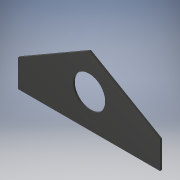
# Autodesk Inventor part: CA01
Saved by Autodesk Inventor 2017 (Build 210142000, 142)
## iProperties
Created: 2019-03-26
Part Number: CA01
Material: ABS Plastic
Document SubType Name: Modeling
Designer: Dell
Density: 1.06 g/cm^3
Appearance: Smooth - Black
Author: Dell
Autodesk Inventor part; units mm, degrees
ref_plane "YZ Plane" through (0, 0, 0) normal (1, 0, 0) x (0, 1, 0)
ref_plane "XZ Plane" through (0, 0, 0) normal (0, 1, 0) x (-1, 0, 0)
ref_plane "XY Plane" through (0, 0, 0) normal (0, 0, 1) x (1, 0, 0)
sketch "Sketch1" plane through (0, 0, 0) normal (0, 0, 1) x (1, 0, 0)
  line L0 (0, 0) -> (525.78, 0)
  line L1 (0, 0) -> (0, 101.6)
  line L2 (0, 101.6) -> (262.89, 253.3796)
  line L3 (262.89, 253.3796) -> (525.78, 101.6)
  line L4 (525.78, 101.6) -> (525.78, 0)
  line L5 (262.89, 246.0473) -> (6.35, 97.9338)
  line L6 (6.35, 97.9338) -> (6.35, 6.35)
  line L7 (6.35, 6.35) -> (519.43, 6.35)
  line L8 (519.43, 6.35) -> (519.43, 97.9338)
  line L9 (519.43, 97.9338) -> (262.89, 246.0473)
  point P0 (262.89, 0)
  dimension "d0" = 525.78
  dimension "d1" = 101.6
  dimension "d2" = 120
  dimension "d3" = 6.35
  constraints: 20 end point, 2 vertical, 1 horizontal, 1 horizontal alignment, 1 midpoint, 1 vertical alignment, 4 other
  measures "d0" distance of L0.start L0.end
  measures "d1" distance of L0.start L1.end
  measures "d2" angle of L1 L2
  measures "d3" distance between parallel lines of L2 L5
extrude "Extrusion1" add sketch "Sketch1" along normal blind 355.6
sketch "Sketch2" plane through (0, 0, 355.6) normal (0, 0, 1) x (1, 0, 0)
  line L0 (262.89, 246.0473) -> (519.43, 97.9338) projected
  line L1 (519.43, 97.9338) -> (519.43, 6.35) projected
  line L2 (519.43, 6.35) -> (6.35, 6.35) projected
  line L3 (6.35, 6.35) -> (6.35, 97.9338) projected
  line L4 (6.35, 97.9338) -> (262.89, 246.0473) projected
  line L5 (0, 0) -> (525.78, 0) projected
  line L6 (525.78, 0) -> (525.78, 101.6) projected
  line L7 (525.78, 101.6) -> (262.89, 253.3796) projected
  line L8 (262.89, 253.3796) -> (0, 101.6) projected
  line L9 (0, 101.6) -> (0, 0) projected
  circle A0 centre (262.89, 121.3796) radius 60
  dimension "d6" = 120
  dimension "d7" = 132
  constraints: 1 centre point, 1 vertical alignment
  measures "d6" diameter of A0
  measures "d7" distance of L7.end A0.centre
extrude "Extrusion2" add sketch "Sketch2" along normal blind 6.35 contours L0 L1 L2 L3 L4 | L9 L8 L7 L6 L5
sketch "Sketch3" plane through (0, 0, 0) normal (0, -1, 0) x (1, 0, 0)
  line L0 (0, 0) -> (525.78, 0) construction
  line L1 (525.78, 0) -> (525.78, 88.9)
  line L2 (525.78, 88.9) -> (0, 88.9) construction
  line L3 (0, 88.9) -> (0, 0) construction
  line L4 (86.36, 21.95) -> (86.36, 66.95) construction
  circle A0 centre (86.36, 44.45) radius 2.3812
  circle A1 centre (86.36, 21.95) radius 2.3812
  circle A2 centre (86.36, 66.95) radius 2.3812
  line L5 (146.36, 49.45) -> (146.36, 29.45) construction
  line L6 (156.36, 66.95) -> (156.36, 21.95) construction
  line L7 (146.36, 29.45) -> (166.36, 29.45) construction
  line L8 (166.36, 49.45) -> (146.36, 49.45) construction
  line L9 (86.36, 66.95) -> (226.36, 66.95) construction
  line L10 (226.36, 21.95) -> (86.36, 21.95) construction
  line L11 (86.36, 44.45) -> (226.36, 44.45) construction
  line L12 (166.36, 29.45) -> (166.36, 49.45) construction
  line L13 (226.36, 66.95) -> (226.36, 21.95) construction
  circle A3 centre (226.36, 66.95) radius 2.3813
  circle A4 centre (226.36, 44.45) radius 2.3813
  circle A5 centre (226.36, 21.95) radius 2.3813
  circle A6 centre (156.36, 39.45) radius 10
  line L14 (0, 0) -> (0, 361.95) projected
  line L15 (525.78, 0) -> (525.78, 361.95) projected
  line L16 (0, 0) -> (525.78, 0) projected
  point P0 (0, 44.45)
  point P1 (146.36, 39.45)
  point P2 (166.36, 39.45)
  point P3 (262.89, 0)
  dimension "d10" = 45
  dimension "d11" = 140
  dimension "d12" = 4.7625
  dimension "d13" = 4.7625
  dimension "d14" = 4.7625
  dimension "d15" = 4.7625
  dimension "d16" = 4.7625
  dimension "d17" = 4.7625
  dimension "d18" = 60
  dimension "d19" = 7.5
  dimension "d20" = 20
  dimension "d21" = 20
  dimension "d22" = 86.36
  dimension "d23" = 88.9
  constraints: 28 end point, 9 midpoint, 6 centre point, 6 parallel, 4 coincident, 3 horizontal alignment, 3 perpendicular, 3 point on line, 1 horizontal, 2 other
  measures "d10" distance of L9.end L10.start
  measures "d11" distance of L9.start L9.end
  measures "d12" diameter of A2
  measures "d13" diameter of A0
  measures "d14" diameter of A1
  measures "d15" diameter of A5
  measures "d16" diameter of A4
  measures "d17" diameter of A3
  measures "d18" distance from line of L11.end L12
  measures "d19" distance between parallel lines of L10 L7
  measures "d20" distance of L8.start L8.end
  measures "d21" distance of L8.end L7.start
  measures "d22" distance between parallel lines of L3 L4
  measures "d23" distance of L2.end L0.start
extrude "Extrusion3" cut sketch "Sketch3" against normal blind 6.35
sketch "Sketch4" plane through (0, 0, 0) normal (0, -1, 0) x (1, 0, 0)
  line L0 (71.36, 0) -> (241.36, 0)
  line L1 (241.36, 0) -> (241.36, 85)
  line L2 (241.36, 85) -> (71.36, 85)
  line L3 (71.36, 85) -> (71.36, 0)
  line L4 (0, 0) -> (525.78, 0) construction
  circle A0 centre (156.36, 39.45) radius 10 construction
  point P0 (156.36, 85)
  dimension "d26" = 170
  dimension "d27" = 85
  constraints: 8 end point, 2 parallel, 1 horizontal, 1 midpoint, 1 perpendicular, 1 point on line, 1 vertical alignment
  measures "d26" distance of L1.end L2.end
  measures "d27" distance of L0.end L1.end
extrude "Extrusion4" cut sketch "Sketch4" against normal blind 6.35
sketch "Sketch5" plane through (0, 0, 361.95) normal (0, -1, 0) x (1, 0, 0)
  line L0 (525.78, -361.95) -> (525.78, 0) projected
  line L1 (0, -361.95) -> (0, 0) projected
  line L2 (525.78, -361.95) -> (0, -361.95)
  line L3 (0, -361.95) -> (0, -124.8833)
  line L4 (0, -124.8833) -> (525.78, -124.8833)
  line L5 (525.78, -124.8833) -> (525.78, -361.95)
  dimension "d30" = 237.0667
  constraints: 8 end point, 2 parallel, 1 horizontal, 1 perpendicular, 1 point on line
  measures "d30" distance between parallel lines of L2 L4
extrude "Extrusion5" cut sketch "Sketch5" against normal through all
sketch "Sketch6" plane through (0, 0, 355.6) normal (0, 0, -1) x (-1, 0, 0)
  line L0 (-519.43, 6.35) -> (-6.35, 6.35) projected
  circle A0 centre (-262.89, 121.3796) radius 60 projected
  line L1 (0, 0) -> (-525.78, 0) projected
  line L2 (-525.78, 0) -> (-525.78, 101.6) projected
  line L3 (-525.78, 101.6) -> (-262.89, 253.3796) projected
  line L4 (-262.89, 253.3796) -> (0, 101.6) projected
  line L5 (0, 101.6) -> (0, 0) projected
extrude "Extrusion6" cut sketch "Sketch6" along normal through all
body "Solid1"
